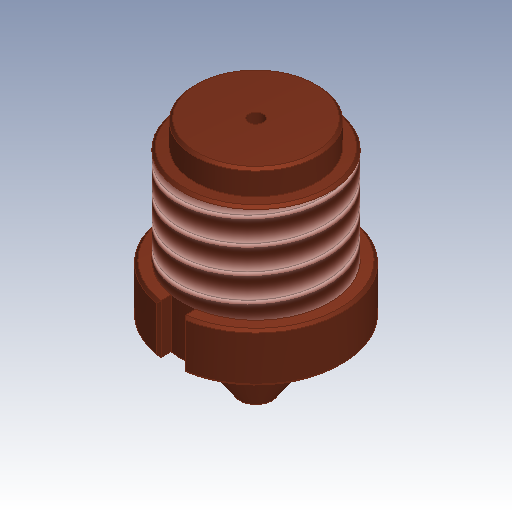
# Autodesk Inventor part: BT011_huenin20_23
Saved by Autodesk Inventor 2023.3 (Build 273359000, 359)
## iProperties
Company: HTBLA Kaindorf
RuleStatus: InUse
Created: 2023-11-27
Part Number: BT011_huenin20_23
Project: Fiberprinter-Hotend
Material: Kupfer
Description: Nozzle
Document SubType Name: Modeling
Designer: huenin20
Density: 8.94 g/cm^3
Appearance: Kupfer - satiniert
Mass: 2.0369 g
Surface Area: 2.39863 cm^2
Volume: 0.227841 cm^3
AfterDocNew0: iProperties-Editor_aufrufen
Author: nicob
Keywords: 2023
Autodesk Inventor part; units mm, degrees
ref_plane "YZ Plane" through (0, 0, 0) normal (1, 0, 0) x (0, 1, 0)
ref_plane "XZ Plane" through (0, 0, 0) normal (0, 1, 0) x (-1, 0, 0)
ref_plane "XY Plane" through (0, 0, 0) normal (0, 0, 1) x (1, 0, 0)
sketch "Skizze3" plane through (0, 0, 0) normal (1, 0, 0) x (0, 1, 0)
  line L0 (0, 0) -> (0, 28.3234)
  line L1 (-3, 4.7135) -> (-3.5, 4.7135)
  line L2 (-3.5, 4.7135) -> (-3.5, 2.7135)
  line L3 (-0.6, 0) -> (-0.3, 0)
  line L4 (-0.3, 0) -> (-0.3, 9.7135)
  line L5 (-0.3, 9.7135) -> (-2.5, 9.7135)
  line L6 (-3, 8.7135) -> (-2.5, 8.7135)
  line L7 (-2.5, 8.7135) -> (-2.5, 9.7135)
  line L8 (-3, 8.7135) -> (-3, 4.7135)
  line L9 (-3.5, 2.7135) -> (-2.5, 2.7135)
  line L10 (-2.5, 2.7135) -> (-0.6, 0)
  point P0 (-1.4, 9.7135)
  dimension "d6" = 2
  dimension "d7" = 7
  dimension "d10" = 0.6
  dimension "d12" = 1.2
  dimension "d13" = 5
  dimension "d14" = 1
  dimension "d15" = 6
  dimension "d16" = 5
  dimension "d20" = 55
  dimension "d31" = 1
  constraints: 23 end point, 3 horizontal, 3 perpendicular, 2 vertical, 1 horizontal alignment, 1 midpoint, 1 parallel
  measures "d6" distance of L1.end L2.end
  measures "d7" diameter of L2 L0
  measures "d10" diameter of L4 L0
  measures "d12" diameter of L3.start L0
  measures "d13" distance from line of point (-1.4, 9.713) L1
  measures "d14" distance of L6.end L5.end
  measures "d15" diameter of L8 L0
  measures "d16" diameter of L7 L0
  measures "d20" angle of L9 L10
  measures "d31" distance of L2.end L9.end
revolve "Umdrehung1" add sketch "Skizze3" angle 360 about axis through (0, 0, 0) along (0, 0, 1)
chamfer "Fase1" distance 0.1 angle 45 4 edges at (0, 3.5, 4.7135) (0, 3.5, 2.7135) (0, 3, 8.7135) (0, 2.5, 9.7135)
fillet "Rundung2" radius 0.2 1 edges at (0, 0.6, 0)
chamfer "Fase2" distance 0.2 angle 45 1 edges at (0, 2.5, 2.7135)
thread "Gewinde1" size "M6x1" class "6g" standard "ISO Metric profile" length 6
sketch "Skizze4" plane through (0, 0, 2.7135) normal (0, 0, -1) x (-1, 0, 0)
  circle A0 centre (0, 0) radius 3.5 projected
  circle A1 centre (0, 0) radius 3 projected
  line L0 (2.958, 0.5) -> (3.4641, 0.5)
  circle A2 centre (0, 0) radius 3.5 projected
  line L1 (4.9, 0) -> (-4.9, 0) projected
  line L2 (2.958, -0.5) -> (3.4641, -0.5)
  point P0 (3.2111, -0.5)
  dimension "d32" = 1
  dimension "d33" = 0.5
  constraints: 4 end point, 4 point on circle, 2 parallel, 1 horizontal, 1 midpoint
  measures "d32" distance between parallel lines of L2 L0
  measures "d33" distance from line of L1 point (3.211, -0.5)
extrude "Extrusion3" cut sketch "Skizze4" against normal through all contours L1 A1 L0 A0 | A0 L2 A1 L1 picked at (3.1345, 0.4447) picked at (3.1345, -0.4447)
chamfer "Fase3" distance 0.1 angle 45 2 edges at (-3.4641, 0.5, 3.7135) (-3.4641, -0.5, 3.7135)
pattern_circular "Runde Anordnung1" count 2 over 360 about axis through (0, 0, 4.8567) along (0, 0, 1) of "Extrusion3", "Fase3"
equation "\"d12\" = 2 * d10"
equation "\"d33\" = 0.5 * d32"
